Autodesk Fusion 360 part; units mm, degrees
(part 4 of 5)
  spline S13 degree 5 poles (13.9862, 0.6207) (13.9784, 0.6259) (13.9629, 0.6363) (13.9395, 0.6518) (13.9082, 0.6724) (13.8691, 0.6978) (13.8299, 0.7229) (13.7907, 0.7477) (13.7514, 0.7723) (13.712, 0.7966) (13.6725, 0.8206) (13.633, 0.8443) (13.5934, 0.8678) (13.5538, 0.8909) (13.514, 0.9138) (13.4743, 0.9364) (13.4344, 0.9587) (13.3946, 0.9807) (13.3546, 1.0024) (13.3146, 1.0239) (13.2746, 1.045) (13.2345, 1.0658) (13.1943, 1.0863) (13.1541, 1.1066) (13.1138, 1.1265) (13.0735, 1.1461) (13.0332, 1.1654) (12.9928, 1.1844) (12.9523, 1.2031) (12.9119, 1.2215) (12.8713, 1.2395) (12.8308, 1.2572) (12.7902, 1.2746) (12.7495, 1.2917) (12.7088, 1.3084) (12.6681, 1.3248) (12.6274, 1.3409) (12.5866, 1.3566) (12.5458, 1.372) (12.505, 1.3871) (12.4641, 1.4018) (12.4233, 1.4161) (12.3824, 1.4301) (12.3414, 1.4437) (12.3005, 1.4569) (12.2595, 1.4698) (12.2186, 1.4823) (12.1776, 1.4944) (12.1366, 1.5062) (12.0956, 1.5175) (12.0545, 1.5285) (12.0135, 1.539) (11.9725, 1.5491) (11.9315, 1.5587) (11.8905, 1.5678) (11.8494, 1.5766) (11.8084, 1.585) (11.7674, 1.5929) (11.7264, 1.6005) (11.6854, 1.6075) (11.6445, 1.614) (11.6035, 1.6199) (11.5626, 1.625) (11.5218, 1.6295) (11.4809, 1.6333) (11.4401, 1.6366) (11.3994, 1.6396) (11.3587, 1.6423) (11.318, 1.6445) (11.2774, 1.6458) (11.237, 1.6456) (11.2048, 1.6439) (11.1807, 1.6416) (11.1647, 1.6395) (11.1567, 1.6383) knots -1 -1 -1 -1 -1 -1 -0.98571429 -0.97142857 -0.95714286 -0.94285714 -0.92857143 -0.91428571 -0.9 -0.88571429 -0.87142857 -0.85714286 -0.84285714 -0.82857143 -0.81428571 -0.8 -0.78571429 -0.77142857 -0.75714286 -0.74285714 -0.72857143 -0.71428571 -0.7 -0.68571429 -0.67142857 -0.65714286 -0.64285714 -0.62857143 -0.61428571 -0.6 -0.58571429 -0.57142857 -0.55714286 -0.54285714 -0.52857143 -0.51428571 -0.5 -0.48571429 -0.47142857 -0.45714286 -0.44285714 -0.42857143 -0.41428571 -0.4 -0.38571429 -0.37142857 -0.35714286 -0.34285714 -0.32857143 -0.31428571 -0.3 -0.28571429 -0.27142857 -0.25714286 -0.24285714 -0.22857143 -0.21428571 -0.2 -0.18571429 -0.17142857 -0.15714286 -0.14285714 -0.12857143 -0.11428571 -0.1 -0.08571429 -0.07142857 -0.05714286 -0.04285714 -0.02857143 -0.01428571 0 0 0 0 0 0
  line L13 (11.1567, 1.6383) -> (10.3893, 1.5263)
  arc A27 (9.2737, 2.2773) -> (10.3893, 1.5263) centre (10.2448, 2.5158) ccw
  arc A28 (9.2737, 2.2773) -> (9.1699, 2.6646) centre (0, 0) ccw
  arc A29 (9.7605, 3.8729) -> (9.1699, 2.6646) centre (10.1302, 2.9437) ccw
  line L14 (9.7605, 3.8729) -> (10.4811, 4.1595)
  spline S14 degree 5 poles (10.4811, 4.1595) (10.4886, 4.1625) (10.5035, 4.1687) (10.5256, 4.1787) (10.5543, 4.1933) (10.5894, 4.2134) (10.6239, 4.2349) (10.658, 4.2571) (10.692, 4.2797) (10.7258, 4.3027) (10.7594, 4.326) (10.7929, 4.3497) (10.826, 4.374) (10.8589, 4.3989) (10.8914, 4.4244) (10.9236, 4.4505) (10.9556, 4.4772) (10.9873, 4.5042) (11.0189, 4.5316) (11.0502, 4.5593) (11.0814, 4.5874) (11.1123, 4.6159) (11.143, 4.6447) (11.1735, 4.674) (11.2038, 4.7036) (11.2338, 4.7336) (11.2637, 4.7639) (11.2933, 4.7946) (11.3227, 4.8256) (11.352, 4.8569) (11.381, 4.8885) (11.4099, 4.9204) (11.4385, 4.9527) (11.4669, 4.9852) (11.4952, 5.0181) (11.5232, 5.0512) (11.551, 5.0847) (11.5787, 5.1184) (11.6061, 5.1524) (11.6334, 5.1867) (11.6604, 5.2213) (11.6873, 5.2561) (11.7139, 5.2912) (11.7404, 5.3266) (11.7666, 5.3622) (11.7927, 5.3981) (11.8186, 5.4343) (11.8443, 5.4707) (11.8698, 5.5073) (11.8951, 5.5442) (11.9202, 5.5813) (11.9451, 5.6187) (11.9698, 5.6563) (11.9943, 5.6942) (12.0186, 5.7323) (12.0427, 5.7706) (12.0667, 5.8092) (12.0904, 5.848) (12.1139, 5.887) (12.1373, 5.9262) (12.1604, 5.9656) (12.1834, 6.0053) (12.2061, 6.0452) (12.2287, 6.0853) (12.251, 6.1256) (12.2732, 6.1661) (12.2952, 6.2069) (12.3169, 6.2478) (12.3385, 6.2889) (12.3599, 6.3303) (12.3811, 6.3718) (12.3979, 6.4052) (12.4104, 6.4304) (12.4186, 6.4472) (12.4228, 6.4556) knots 0 0 0 0 0 0 0.01428571 0.02857143 0.04285714 0.05714286 0.07142857 0.08571429 0.1 0.11428571 0.12857143 0.14285714 0.15714286 0.17142857 0.18571429 0.2 0.21428571 0.22857143 0.24285714 0.25714286 0.27142857 0.28571429 0.3 0.31428571 0.32857143 0.34285714 0.35714286 0.37142857 0.38571429 0.4 0.41428571 0.42857143 0.44285714 0.45714286 0.47142857 0.48571429 0.5 0.51428571 0.52857143 0.54285714 0.55714286 0.57142857 0.58571429 0.6 0.61428571 0.62857143 0.64285714 0.65714286 0.67142857 0.68571429 0.7 0.71428571 0.72857143 0.74285714 0.75714286 0.77142857 0.78571429 0.8 0.81428571 0.82857143 0.84285714 0.85714286 0.87142857 0.88571429 0.9 0.91428571 0.92857143 0.94285714 0.95714286 0.97142857 0.98571429 1 1 1 1 1 1
  arc A30 (12.4228, 6.4556) -> (11.8021, 7.5307) centre (0, 0) ccw
  spline S15 degree 5 poles (11.8021, 7.5307) (11.7927, 7.5313) (11.774, 7.5325) (11.746, 7.5342) (11.7087, 7.5364) (11.6621, 7.5388) (11.6156, 7.541) (11.5692, 7.5429) (11.5229, 7.5445) (11.4766, 7.5458) (11.4305, 7.5469) (11.3844, 7.5477) (11.3384, 7.5482) (11.2924, 7.5484) (11.2466, 7.5484) (11.2009, 7.5481) (11.1552, 7.5475) (11.1097, 7.5466) (11.0642, 7.5454) (11.0189, 7.544) (10.9736, 7.5423) (10.9285, 7.5403) (10.8834, 7.538) (10.8385, 7.5354) (10.7937, 7.5325) (10.7489, 7.5293) (10.7044, 7.5259) (10.6599, 7.5221) (10.6155, 7.5181) (10.5713, 7.5137) (10.5271, 7.5091) (10.4832, 7.5042) (10.4393, 7.4989) (10.3956, 7.4934) (10.352, 7.4876) (10.3085, 7.4814) (10.2652, 7.475) (10.222, 7.4682) (10.179, 7.4611) (10.1361, 7.4538) (10.0934, 7.4461) (10.0508, 7.438) (10.0084, 7.4297) (9.9662, 7.421) (9.9241, 7.412) (9.8822, 7.4027) (9.8404, 7.393) (9.7989, 7.383) (9.7575, 7.3727) (9.7163, 7.362) (9.6753, 7.351) (9.6345, 7.3396) (9.594, 7.3278) (9.5536, 7.3156) (9.5135, 7.303) (9.4736, 7.2901) (9.4339, 7.2768) (9.3944, 7.2632) (9.3551, 7.2492) (9.3161, 7.2349) (9.2774, 7.22) (9.239, 7.2046) (9.201, 7.1886) (9.1634, 7.172) (9.1261, 7.1549) (9.0891, 7.1374) (9.0523, 7.1196) (9.0157, 7.1016) (8.9794, 7.0831) (8.9437, 7.064) (8.9087, 7.0436) (8.8816, 7.0261) (8.862, 7.012) (8.8491, 7.0022) (8.8428, 6.9972) knots -1 -1 -1 -1 -1 -1 -0.98571429 -0.97142857 -0.95714286 -0.94285714 -0.92857143 -0.91428571 -0.9 -0.88571429 -0.87142857 -0.85714286 -0.84285714 -0.82857143 -0.81428571 -0.8 -0.78571429 -0.77142857 -0.75714286 -0.74285714 -0.72857143 -0.71428571 -0.7 -0.68571429 -0.67142857 -0.65714286 -0.64285714 -0.62857143 -0.61428571 -0.6 -0.58571429 -0.57142857 -0.55714286 -0.54285714 -0.52857143 -0.51428571 -0.5 -0.48571429 -0.47142857 -0.45714286 -0.44285714 -0.42857143 -0.41428571 -0.4 -0.38571429 -0.37142857 -0.35714286 -0.34285714 -0.32857143 -0.31428571 -0.3 -0.28571429 -0.27142857 -0.25714286 -0.24285714 -0.22857143 -0.21428571 -0.2 -0.18571429 -0.17142857 -0.15714286 -0.14285714 -0.12857143 -0.11428571 -0.1 -0.08571429 -0.07142857 -0.05714286 -0.04285714 -0.02857143 -0.01428571 0 0 0 0 0 0
  line L15 (8.8428, 6.9972) -> (8.2343, 6.5164)
  arc A31 (6.8926, 6.609) -> (8.2343, 6.5164) centre (7.6144, 7.3011) ccw
  arc A32 (6.8926, 6.609) -> (6.609, 6.8926) centre (0, 0) ccw
  arc A33 (6.5164, 8.2343) -> (6.609, 6.8926) centre (7.3011, 7.6144) ccw
  line L16 (6.5164, 8.2343) -> (6.9972, 8.8428)
  spline S16 degree 5 poles (6.9972, 8.8428) (7.0022, 8.8491) (7.012, 8.862) (7.0261, 8.8816) (7.0436, 8.9087) (7.064, 8.9437) (7.0831, 8.9794) (7.1016, 9.0157) (7.1196, 9.0523) (7.1374, 9.0891) (7.1549, 9.1261) (7.172, 9.1634) (7.1886, 9.201) (7.2046, 9.239) (7.22, 9.2774) (7.2349, 9.3161) (7.2492, 9.3551) (7.2632, 9.3944) (7.2768, 9.4339) (7.2901, 9.4736) (7.303, 9.5135) (7.3156, 9.5536) (7.3278, 9.594) (7.3396, 9.6345) (7.351, 9.6753) (7.362, 9.7163) (7.3727, 9.7575) (7.383, 9.7989) (7.393, 9.8404) (7.4027, 9.8822) (7.412, 9.9241) (7.421, 9.9662) (7.4297, 10.0084) (7.438, 10.0508) (7.4461, 10.0934) (7.4538, 10.1361) (7.4611, 10.179) (7.4682, 10.222) (7.475, 10.2652) (7.4814, 10.3085) (7.4876, 10.352) (7.4934, 10.3956) (7.4989, 10.4393) (7.5042, 10.4832) (7.5091, 10.5271) (7.5137, 10.5713) (7.5181, 10.6155) (7.5221, 10.6599) (7.5259, 10.7044) (7.5293, 10.7489) (7.5325, 10.7937) (7.5354, 10.8385) (7.538, 10.8834) (7.5403, 10.9285) (7.5423, 10.9736) (7.544, 11.0189) (7.5454, 11.0642) (7.5466, 11.1097) (7.5475, 11.1552) (7.5481, 11.2009) (7.5484, 11.2466) (7.5484, 11.2924) (7.5482, 11.3384) (7.5477, 11.3844) (7.5469, 11.4305) (7.5458, 11.4766) (7.5445, 11.5229) (7.5429, 11.5692) (7.541, 11.6156) (7.5388, 11.6621) (7.5364, 11.7087) (7.5342, 11.746) (7.5325, 11.774) (7.5313, 11.7927) (7.5307, 11.8021) knots 0 0 0 0 0 0 0.01428571 0.02857143 0.04285714 0.05714286 0.07142857 0.08571429 0.1 0.11428571 0.12857143 0.14285714 0.15714286 0.17142857 0.18571429 0.2 0.21428571 0.22857143 0.24285714 0.25714286 0.27142857 0.28571429 0.3 0.31428571 0.32857143 0.34285714 0.35714286 0.37142857 0.38571429 0.4 0.41428571 0.42857143 0.44285714 0.45714286 0.47142857 0.48571429 0.5 0.51428571 0.52857143 0.54285714 0.55714286 0.57142857 0.58571429 0.6 0.61428571 0.62857143 0.64285714 0.65714286 0.67142857 0.68571429 0.7 0.71428571 0.72857143 0.74285714 0.75714286 0.77142857 0.78571429 0.8 0.81428571 0.82857143 0.84285714 0.85714286 0.87142857 0.88571429 0.9 0.91428571 0.92857143 0.94285714 0.95714286 0.97142857 0.98571429 1 1 1 1 1 1
  arc A34 (7.5307, 11.8021) -> (6.4556, 12.4228) centre (0, 0) ccw
  spline S17 degree 5 poles (6.4556, 12.4228) (6.4472, 12.4186) (6.4304, 12.4104) (6.4052, 12.3979) (6.3718, 12.3811) (6.3303, 12.3599) (6.2889, 12.3385) (6.2478, 12.3169) (6.2069, 12.2952) (6.1661, 12.2732) (6.1256, 12.251) (6.0853, 12.2287) (6.0452, 12.2061) (6.0053, 12.1834) (5.9656, 12.1604) (5.9262, 12.1373) (5.887, 12.1139) (5.848, 12.0904) (5.8092, 12.0667) (5.7706, 12.0427) (5.7323, 12.0186) (5.6942, 11.9943) (5.6563, 11.9698) (5.6187, 11.9451) (5.5813, 11.9202) (5.5442, 11.8951) (5.5073, 11.8698) (5.4707, 11.8443) (5.4343, 11.8186) (5.3981, 11.7927) (5.3622, 11.7666) (5.3266, 11.7404) (5.2912, 11.7139) (5.2561, 11.6873) (5.2213, 11.6604) (5.1867, 11.6334) (5.1524, 11.6061) (5.1184, 11.5787) (5.0847, 11.551) (5.0512, 11.5232) (5.0181, 11.4952) (4.9852, 11.4669) (4.9527, 11.4385) (4.9204, 11.4099) (4.8885, 11.381) (4.8569, 11.352) (4.8256, 11.3227) (4.7946, 11.2933) (4.7639, 11.2637) (4.7336, 11.2338) (4.7036, 11.2038) (4.674, 11.1735) (4.6447, 11.143) (4.6159, 11.1123) (4.5874, 11.0814) (4.5593, 11.0502) (4.5316, 11.0189) (4.5042, 10.9873) (4.4772, 10.9556) (4.4505, 10.9236) (4.4244, 10.8914) (4.3989, 10.8589) (4.374, 10.826) (4.3497, 10.7929) (4.326, 10.7594) (4.3027, 10.7258) (4.2797, 10.692) (4.2571, 10.658) (4.2349, 10.6239) (4.2134, 10.5894) (4.1933, 10.5543) (4.1787, 10.5256) (4.1687, 10.5035) (4.1625, 10.4886) (4.1595, 10.4811) knots -1 -1 -1 -1 -1 -1 -0.98571429 -0.97142857 -0.95714286 -0.94285714 -0.92857143 -0.91428571 -0.9 -0.88571429 -0.87142857 -0.85714286 -0.84285714 -0.82857143 -0.81428571 -0.8 -0.78571429 -0.77142857 -0.75714286 -0.74285714 -0.72857143 -0.71428571 -0.7 -0.68571429 -0.67142857 -0.65714286 -0.64285714 -0.62857143 -0.61428571 -0.6 -0.58571429 -0.57142857 -0.55714286 -0.54285714 -0.52857143 -0.51428571 -0.5 -0.48571429 -0.47142857 -0.45714286 -0.44285714 -0.42857143 -0.41428571 -0.4 -0.38571429 -0.37142857 -0.35714286 -0.34285714 -0.32857143 -0.31428571 -0.3 -0.28571429 -0.27142857 -0.25714286 -0.24285714 -0.22857143 -0.21428571 -0.2 -0.18571429 -0.17142857 -0.15714286 -0.14285714 -0.12857143 -0.11428571 -0.1 -0.08571429 -0.07142857 -0.05714286 -0.04285714 -0.02857143 -0.01428571 0 0 0 0 0 0
  line L17 (4.1595, 10.4811) -> (3.8729, 9.7605)
  arc A35 (2.6646, 9.1699) -> (3.8729, 9.7605) centre (2.9437, 10.1302) ccw
  arc A36 (2.6646, 9.1699) -> (2.2773, 9.2737) centre (0, 0) ccw
  arc A37 (1.5263, 10.3893) -> (2.2773, 9.2737) centre (2.5158, 10.2448) ccw
  line L18 (1.5263, 10.3893) -> (1.6383, 11.1567)
  spline S18 degree 5 poles (1.6383, 11.1567) (1.6395, 11.1647) (1.6416, 11.1807) (1.6439, 11.2048) (1.6456, 11.237) (1.6458, 11.2774) (1.6445, 11.318) (1.6423, 11.3587) (1.6396, 11.3994) (1.6366, 11.4401) (1.6333, 11.4809) (1.6295, 11.5218) (1.625, 11.5626) (1.6199, 11.6035) (1.614, 11.6445) (1.6075, 11.6854) (1.6005, 11.7264) (1.5929, 11.7674) (1.585, 11.8084) (1.5766, 11.8494) (1.5678, 11.8905) (1.5587, 11.9315) (1.5491, 11.9725) (1.539, 12.0135) (1.5285, 12.0545) (1.5175, 12.0956) (1.5062, 12.1366) (1.4944, 12.1776) (1.4823, 12.2186) (1.4698, 12.2595) (1.4569, 12.3005) (1.4437, 12.3414) (1.4301, 12.3824) (1.4161, 12.4233) (1.4018, 12.4641) (1.3871, 12.505) (1.372, 12.5458) (1.3566, 12.5866) (1.3409, 12.6274) (1.3248, 12.6681) (1.3084, 12.7088) (1.2917, 12.7495) (1.2746, 12.7902) (1.2572, 12.8308) (1.2395, 12.8713) (1.2215, 12.9119) (1.2031, 12.9523) (1.1844, 12.9928) (1.1654, 13.0332) (1.1461, 13.0735) (1.1265, 13.1138) (1.1066, 13.1541) (1.0863, 13.1943) (1.0658, 13.2345) (1.045, 13.2746) (1.0239, 13.3146) (1.0024, 13.3546) (0.9807, 13.3946) (0.9587, 13.4344) (0.9364, 13.4743) (0.9138, 13.514) (0.8909, 13.5538) (0.8678, 13.5934) (0.8443, 13.633) (0.8206, 13.6725) (0.7966, 13.712) (0.7723, 13.7514) (0.7477, 13.7907) (0.7229, 13.8299) (0.6978, 13.8691) (0.6724, 13.9082) (0.6518, 13.9395) (0.6363, 13.9629) (0.6259, 13.9784) (0.6207, 13.9862) knots 0 0 0 0 0 0 0.01428571 0.02857143 0.04285714 0.05714286 0.07142857 0.08571429 0.1 0.11428571 0.12857143 0.14285714 0.15714286 0.17142857 0.18571429 0.2 0.21428571 0.22857143 0.24285714 0.25714286 0.27142857 0.28571429 0.3 0.31428571 0.32857143 0.34285714 0.35714286 0.37142857 0.38571429 0.4 0.41428571 0.42857143 0.44285714 0.45714286 0.47142857 0.48571429 0.5 0.51428571 0.52857143 0.54285714 0.55714286 0.57142857 0.58571429 0.6 0.61428571 0.62857143 0.64285714 0.65714286 0.67142857 0.68571429 0.7 0.71428571 0.72857143 0.74285714 0.75714286 0.77142857 0.78571429 0.8 0.81428571 0.82857143 0.84285714 0.85714286 0.87142857 0.88571429 0.9 0.91428571 0.92857143 0.94285714 0.95714286 0.97142857 0.98571429 1 1 1 1 1 1
  arc A38 (0.6207, 13.9862) -> (-0.6207, 13.9862) centre (0, 0) ccw
  spline S19 degree 5 poles (-0.6207, 13.9862) (-0.6259, 13.9784) (-0.6363, 13.9629) (-0.6518, 13.9395) (-0.6724, 13.9082) (-0.6978, 13.8691) (-0.7229, 13.8299) (-0.7477, 13.7907) (-0.7723, 13.7514) (-0.7966, 13.712) (-0.8206, 13.6725) (-0.8443, 13.633) (-0.8678, 13.5934) (-0.8909, 13.5538) (-0.9138, 13.514) (-0.9364, 13.4743) (-0.9587, 13.4344) (-0.9807, 13.3946) (-1.0024, 13.3546) (-1.0239, 13.3146) (-1.045, 13.2746) (-1.0658, 13.2345) (-1.0863, 13.1943) (-1.1066, 13.1541) (-1.1265, 13.1138) (-1.1461, 13.0735) (-1.1654, 13.0332) (-1.1844, 12.9928) (-1.2031, 12.9523) (-1.2215, 12.9119) (-1.2395, 12.8713) (-1.2572, 12.8308) (-1.2746, 12.7902) (-1.2917, 12.7495) (-1.3084, 12.7088) (-1.3248, 12.6681) (-1.3409, 12.6274) (-1.3566, 12.5866) (-1.372, 12.5458) (-1.3871, 12.505) (-1.4018, 12.4641) (-1.4161, 12.4233) (-1.4301, 12.3824) (-1.4437, 12.3414) (-1.4569, 12.3005) (-1.4698, 12.2595) (-1.4823, 12.2186) (-1.4944, 12.1776) (-1.5062, 12.1366) (-1.5175, 12.0956) (-1.5285, 12.0545) (-1.539, 12.0135) (-1.5491, 11.9725) (-1.5587, 11.9315) (-1.5678, 11.8905) (-1.5766, 11.8494) (-1.585, 11.8084) (-1.5929, 11.7674) (-1.6005, 11.7264) (-1.6075, 11.6854) (-1.614, 11.6445) (-1.6199, 11.6035) (-1.625, 11.5626) (-1.6295, 11.5218) (-1.6333, 11.4809) (-1.6366, 11.4401) (-1.6396, 11.3994) (-1.6423, 11.3587) (-1.6445, 11.318) (-1.6458, 11.2774) (-1.6456, 11.237) (-1.6439, 11.2048) (-1.6416, 11.1807) (-1.6395, 11.1647) (-1.6383, 11.1567) knots -1 -1 -1 -1 -1 -1 -0.98571429 -0.97142857 -0.95714286 -0.94285714 -0.92857143 -0.91428571 -0.9 -0.88571429 -0.87142857 -0.85714286 -0.84285714 -0.82857143 -0.81428571 -0.8 -0.78571429 -0.77142857 -0.75714286 -0.74285714 -0.72857143 -0.71428571 -0.7 -0.68571429 -0.67142857 -0.65714286 -0.64285714 -0.62857143 -0.61428571 -0.6 -0.58571429 -0.57142857 -0.55714286 -0.54285714 -0.52857143 -0.51428571 -0.5 -0.48571429 -0.47142857 -0.45714286 -0.44285714 -0.42857143 -0.41428571 -0.4 -0.38571429 -0.37142857 -0.35714286 -0.34285714 -0.32857143 -0.31428571 -0.3 -0.28571429 -0.27142857 -0.25714286 -0.24285714 -0.22857143 -0.21428571 -0.2 -0.18571429 -0.17142857 -0.15714286 -0.14285714 -0.12857143 -0.11428571 -0.1 -0.08571429 -0.07142857 -0.05714286 -0.04285714 -0.02857143 -0.01428571 0 0 0 0 0 0
  line L19 (-1.6383, 11.1567) -> (-1.5263, 10.3893)
  arc A39 (-2.2773, 9.2737) -> (-1.5263, 10.3893) centre (-2.5158, 10.2448) ccw
  arc A40 (-2.2773, 9.2737) -> (-2.6646, 9.1699) centre (0, 0) ccw
  arc A41 (-3.8729, 9.7605) -> (-2.6646, 9.1699) centre (-2.9437, 10.1302) ccw
  line L20 (-3.8729, 9.7605) -> (-4.1595, 10.4811)
  spline S20 degree 5 poles (-4.1595, 10.4811) (-4.1625, 10.4886) (-4.1687, 10.5035) (-4.1787, 10.5256) (-4.1933, 10.5543) (-4.2134, 10.5894) (-4.2349, 10.6239) (-4.2571, 10.658) (-4.2797, 10.692) (-4.3027, 10.7258) (-4.326, 10.7594) (-4.3497, 10.7929) (-4.374, 10.826) (-4.3989, 10.8589) (-4.4244, 10.8914) (-4.4505, 10.9236) (-4.4772, 10.9556) (-4.5042, 10.9873) (-4.5316, 11.0189) (-4.5593, 11.0502) (-4.5874, 11.0814) (-4.6159, 11.1123) (-4.6447, 11.143) (-4.674, 11.1735) (-4.7036, 11.2038) (-4.7336, 11.2338) (-4.7639, 11.2637) (-4.7946, 11.2933) (-4.8256, 11.3227) (-4.8569, 11.352) (-4.8885, 11.381) (-4.9204, 11.4099) (-4.9527, 11.4385) (-4.9852, 11.4669) (-5.0181, 11.4952) (-5.0512, 11.5232) (-5.0847, 11.551) (-5.1184, 11.5787) (-5.1524, 11.6061) (-5.1867, 11.6334) (-5.2213, 11.6604) (-5.2561, 11.6873) (-5.2912, 11.7139) (-5.3266, 11.7404) (-5.3622, 11.7666) (-5.3981, 11.7927) (-5.4343, 11.8186) (-5.4707, 11.8443) (-5.5073, 11.8698) (-5.5442, 11.8951) (-5.5813, 11.9202) (-5.6187, 11.9451) (-5.6563, 11.9698) (-5.6942, 11.9943) (-5.7323, 12.0186) (-5.7706, 12.0427) (-5.8092, 12.0667) (-5.848, 12.0904) (-5.887, 12.1139) (-5.9262, 12.1373) (-5.9656, 12.1604) (-6.0053, 12.1834) (-6.0452, 12.2061) (-6.0853, 12.2287) (-6.1256, 12.251) (-6.1661, 12.2732) (-6.2069, 12.2952) (-6.2478, 12.3169) (-6.2889, 12.3385) (-6.3303, 12.3599) (-6.3718, 12.3811) (-6.4052, 12.3979) (-6.4304, 12.4104) (-6.4472, 12.4186) (-6.4556, 12.4228) knots 0 0 0 0 0 0 0.01428571 0.02857143 0.04285714 0.05714286 0.07142857 0.08571429 0.1 0.11428571 0.12857143 0.14285714 0.15714286 0.17142857 0.18571429 0.2 0.21428571 0.22857143 0.24285714 0.25714286 0.27142857 0.28571429 0.3 0.31428571 0.32857143 0.34285714 0.35714286 0.37142857 0.38571429 0.4 0.41428571 0.42857143 0.44285714 0.45714286 0.47142857 0.48571429 0.5 0.51428571 0.52857143 0.54285714 0.55714286 0.57142857 0.58571429 0.6 0.61428571 0.62857143 0.64285714 0.65714286 0.67142857 0.68571429 0.7 0.71428571 0.72857143 0.74285714 0.75714286 0.77142857 0.78571429 0.8 0.81428571 0.82857143 0.84285714 0.85714286 0.87142857 0.88571429 0.9 0.91428571 0.92857143 0.94285714 0.95714286 0.97142857 0.98571429 1 1 1 1 1 1
  arc A42 (-6.4556, 12.4228) -> (-7.5307, 11.8021) centre (0, 0) ccw
  spline S21 degree 5 poles (-7.5307, 11.8021) (-7.5313, 11.7927) (-7.5325, 11.774) (-7.5342, 11.746) (-7.5364, 11.7087) (-7.5388, 11.6621) (-7.541, 11.6156) (-7.5429, 11.5692) (-7.5445, 11.5229) (-7.5458, 11.4766) (-7.5469, 11.4305) (-7.5477, 11.3844) (-7.5482, 11.3384) (-7.5484, 11.2924) (-7.5484, 11.2466) (-7.5481, 11.2009) (-7.5475, 11.1552) (-7.5466, 11.1097) (-7.5454, 11.0642) (-7.544, 11.0189) (-7.5423, 10.9736) (-7.5403, 10.9285) (-7.538, 10.8834) (-7.5354, 10.8385) (-7.5325, 10.7937) (-7.5293, 10.7489) (-7.5259, 10.7044) (-7.5221, 10.6599) (-7.5181, 10.6155) (-7.5137, 10.5713) (-7.5091, 10.5271) (-7.5042, 10.4832) (-7.4989, 10.4393) (-7.4934, 10.3956) (-7.4876, 10.352) (-7.4814, 10.3085) (-7.475, 10.2652) (-7.4682, 10.222) (-7.4611, 10.179) (-7.4538, 10.1361) (-7.4461, 10.0934) (-7.438, 10.0508) (-7.4297, 10.0084) (-7.421, 9.9662) (-7.412, 9.9241) (-7.4027, 9.8822) (-7.393, 9.8404) (-7.383, 9.7989) (-7.3727, 9.7575) (-7.362, 9.7163) (-7.351, 9.6753) (-7.3396, 9.6345) (-7.3278, 9.594) (-7.3156, 9.5536) (-7.303, 9.5135) (-7.2901, 9.4736) (-7.2768, 9.4339) (-7.2632, 9.3944) (-7.2492, 9.3551) (-7.2349, 9.3161) (-7.22, 9.2774) (-7.2046, 9.239) (-7.1886, 9.201) (-7.172, 9.1634) (-7.1549, 9.1261) (-7.1374, 9.0891) (-7.1196, 9.0523) (-7.1016, 9.0157) (-7.0831, 8.9794) (-7.064, 8.9437) (-7.0436, 8.9087) (-7.0261, 8.8816) (-7.012, 8.862) (-7.0022, 8.8491) (-6.9972, 8.8428) knots -1 -1 -1 -1 -1 -1 -0.98571429 -0.97142857 -0.95714286 -0.94285714 -0.92857143 -0.91428571 -0.9 -0.88571429 -0.87142857 -0.85714286 -0.84285714 -0.82857143 -0.81428571 -0.8 -0.78571429 -0.77142857 -0.75714286 -0.74285714 -0.72857143 -0.71428571 -0.7 -0.68571429 -0.67142857 -0.65714286 -0.64285714 -0.62857143 -0.61428571 -0.6 -0.58571429 -0.57142857 -0.55714286 -0.54285714 -0.52857143 -0.51428571 -0.5 -0.48571429 -0.47142857 -0.45714286 -0.44285714 -0.42857143 -0.41428571 -0.4 -0.38571429 -0.37142857 -0.35714286 -0.34285714 -0.32857143 -0.31428571 -0.3 -0.28571429 -0.27142857 -0.25714286 -0.24285714 -0.22857143 -0.21428571 -0.2 -0.18571429 -0.17142857 -0.15714286 -0.14285714 -0.12857143 -0.11428571 -0.1 -0.08571429 -0.07142857 -0.05714286 -0.04285714 -0.02857143 -0.01428571 0 0 0 0 0 0
  line L21 (-6.9972, 8.8428) -> (-6.5164, 8.2343)
  arc A43 (-6.609, 6.8926) -> (-6.5164, 8.2343) centre (-7.3011, 7.6144) ccw
  arc A44 (-6.609, 6.8926) -> (-6.8926, 6.609) centre (0, 0) ccw
  arc A45 (-8.2343, 6.5164) -> (-6.8926, 6.609) centre (-7.6144, 7.3011) ccw
  line L22 (-8.2343, 6.5164) -> (-8.8428, 6.9972)
  spline S22 degree 5 poles (-8.8428, 6.9972) (-8.8491, 7.0022) (-8.862, 7.012) (-8.8816, 7.0261) (-8.9087, 7.0436) (-8.9437, 7.064) (-8.9794, 7.0831) (-9.0157, 7.1016) (-9.0523, 7.1196) (-9.0891, 7.1374) (-9.1261, 7.1549) (-9.1634, 7.172) (-9.201, 7.1886) (-9.239, 7.2046) (-9.2774, 7.22) (-9.3161, 7.2349) (-9.3551, 7.2492) (-9.3944, 7.2632) (-9.4339, 7.2768) (-9.4736, 7.2901) (-9.5135, 7.303) (-9.5536, 7.3156) (-9.594, 7.3278) (-9.6345, 7.3396) (-9.6753, 7.351) (-9.7163, 7.362) (-9.7575, 7.3727) (-9.7989, 7.383) (-9.8404, 7.393) (-9.8822, 7.4027) (-9.9241, 7.412) (-9.9662, 7.421) (-10.0084, 7.4297) (-10.0508, 7.438) (-10.0934, 7.4461) (-10.1361, 7.4538) (-10.179, 7.4611) (-10.222, 7.4682) (-10.2652, 7.475) (-10.3085, 7.4814) (-10.352, 7.4876) (-10.3956, 7.4934) (-10.4393, 7.4989) (-10.4832, 7.5042) (-10.5271, 7.5091) (-10.5713, 7.5137) (-10.6155, 7.5181) (-10.6599, 7.5221) (-10.7044, 7.5259) (-10.7489, 7.5293) (-10.7937, 7.5325) (-10.8385, 7.5354) (-10.8834, 7.538) (-10.9285, 7.5403) (-10.9736, 7.5423) (-11.0189, 7.544) (-11.0642, 7.5454) (-11.1097, 7.5466) (-11.1552, 7.5475) (-11.2009, 7.5481) (-11.2466, 7.5484) (-11.2924, 7.5484) (-11.3384, 7.5482) (-11.3844, 7.5477) (-11.4305, 7.5469) (-11.4766, 7.5458) (-11.5229, 7.5445) (-11.5692, 7.5429) (-11.6156, 7.541) (-11.6621, 7.5388) (-11.7087, 7.5364) (-11.746, 7.5342) (-11.774, 7.5325) (-11.7927, 7.5313) (-11.8021, 7.5307) knots 0 0 0 0 0 0 0.01428571 0.02857143 0.04285714 0.05714286 0.07142857 0.08571429 0.1 0.11428571 0.12857143 0.14285714 0.15714286 0.17142857 0.18571429 0.2 0.21428571 0.22857143 0.24285714 0.25714286 0.27142857 0.28571429 0.3 0.31428571 0.32857143 0.34285714 0.35714286 0.37142857 0.38571429 0.4 0.41428571 0.42857143 0.44285714 0.45714286 0.47142857 0.48571429 0.5 0.51428571 0.52857143 0.54285714 0.55714286 0.57142857 0.58571429 0.6 0.61428571 0.62857143 0.64285714 0.65714286 0.67142857 0.68571429 0.7 0.71428571 0.72857143 0.74285714 0.75714286 0.77142857 0.78571429 0.8 0.81428571 0.82857143 0.84285714 0.85714286 0.87142857 0.88571429 0.9 0.91428571 0.92857143 0.94285714 0.95714286 0.97142857 0.98571429 1 1 1 1 1 1
  arc A46 (-11.8021, 7.5307) -> (-12.4228, 6.4556) centre (0, 0) ccw
  spline S23 degree 5 poles (-12.4228, 6.4556) (-12.4186, 6.4472) (-12.4104, 6.4304) (-12.3979, 6.4052) (-12.3811, 6.3718) (-12.3599, 6.3303) (-12.3385, 6.2889) (-12.3169, 6.2478) (-12.2952, 6.2069) (-12.2732, 6.1661) (-12.251, 6.1256) (-12.2287, 6.0853) (-12.2061, 6.0452) (-12.1834, 6.0053) (-12.1604, 5.9656) (-12.1373, 5.9262) (-12.1139, 5.887) (-12.0904, 5.848) (-12.0667, 5.8092) (-12.0427, 5.7706) (-12.0186, 5.7323) (-11.9943, 5.6942) (-11.9698, 5.6563) (-11.9451, 5.6187) (-11.9202, 5.5813) (-11.8951, 5.5442) (-11.8698, 5.5073) (-11.8443, 5.4707) (-11.8186, 5.4343) (-11.7927, 5.3981) (-11.7666, 5.3622) (-11.7404, 5.3266) (-11.7139, 5.2912) (-11.6873, 5.2561) (-11.6604, 5.2213) (-11.6334, 5.1867) (-11.6061, 5.1524) (-11.5787, 5.1184) (-11.551, 5.0847) (-11.5232, 5.0512) (-11.4952, 5.0181) (-11.4669, 4.9852) (-11.4385, 4.9527) (-11.4099, 4.9204) (-11.381, 4.8885) (-11.352, 4.8569) (-11.3227, 4.8256) (-11.2933, 4.7946) (-11.2637, 4.7639) (-11.2338, 4.7336) (-11.2038, 4.7036) (-11.1735, 4.674) (-11.143, 4.6447) (-11.1123, 4.6159) (-11.0814, 4.5874) (-11.0502, 4.5593) (-11.0189, 4.5316) (-10.9873, 4.5042) (-10.9556, 4.4772) (-10.9236, 4.4505) (-10.8914, 4.4244) (-10.8589, 4.3989) (-10.826, 4.374) (-10.7929, 4.3497) (-10.7594, 4.326) (-10.7258, 4.3027) (-10.692, 4.2797) (-10.658, 4.2571) (-10.6239, 4.2349) (-10.5894, 4.2134) (-10.5543, 4.1933) (-10.5256, 4.1787) (-10.5035, 4.1687) (-10.4886, 4.1625) (-10.4811, 4.1595) knots -1 -1 -1 -1 -1 -1 -0.98571429 -0.97142857 -0.95714286 -0.94285714 -0.92857143 -0.91428571 -0.9 -0.88571429 -0.87142857 -0.85714286 -0.84285714 -0.82857143 -0.81428571 -0.8 -0.78571429 -0.77142857 -0.75714286 -0.74285714 -0.72857143 -0.71428571 -0.7 -0.68571429 -0.67142857 -0.65714286 -0.64285714 -0.62857143 -0.61428571 -0.6 -0.58571429 -0.57142857 -0.55714286 -0.54285714 -0.52857143 -0.51428571 -0.5 -0.48571429 -0.47142857 -0.45714286 -0.44285714 -0.42857143 -0.41428571 -0.4 -0.38571429 -0.37142857 -0.35714286 -0.34285714 -0.32857143 -0.31428571 -0.3 -0.28571429 -0.27142857 -0.25714286 -0.24285714 -0.22857143 -0.21428571 -0.2 -0.18571429 -0.17142857 -0.15714286 -0.14285714 -0.12857143 -0.11428571 -0.1 -0.08571429 -0.07142857 -0.05714286 -0.04285714 -0.02857143 -0.01428571 0 0 0 0 0 0
  line L23 (-10.4811, 4.1595) -> (-9.7605, 3.8729)
  arc A47 (-9.1699, 2.6646) -> (-9.7605, 3.8729) centre (-10.1302, 2.9437) ccw
  circle A48 centre (0, 0) radius 2.5
  circle A49 centre (0, 0) radius 9.5492
  circle A50 centre (0, 0) radius 15.4387
  line L24 (6.8926, -6.609) -> (10.9038, -10.9299)
  line L25 (-2.6646, 9.1699) -> (-4.5624, 14.7492)
  constraint concentric A0 A49
  constraint coincident A16.end A49
  constraint concentric A49 A50
  constraint coincident A20.end A21.end
  constraint coincident A50 L24.end
  constraint coincident A40.end A41.end
  constraint coincident A50 L25.end
extrude "Extrude3" cut sketch "Sketch1 (2)" against normal blind 8 contours A21 L10 S10 A22 S11 L11 A23 A24 A25 L12 S12 A26 S13 L13 A27 A28 A29 L14 S14 A30 S15 L15 A31 A32 A33 L16 S16 A34 S17 L17 A35 A36 A37 L18 S18 A38 S19 L19 A39 A40 A49 A50 L24 L25 | A37 L18 S18 A38 S19 L19 A39 A49 | A33 L16 S16 A34 S17 L17 A35 A49 | A21 L10 S10 A22 S11 L11 A23 A49 | A29 L14 S14 A30 S15 L15 A31 A49 | A25 L12 S12 A26 S13 L13 A27 A49 in component "Spur Gear (12 teeth)"
sketch "Sketch2 (2)" plane through (-81.2627, 96.8451, -716.9768) normal (0.111619, -0.133022, 0.984808) x (0.766044, 0.642788, 0)
  arc A0 (-12.2773, -144.5539) -> (-12.2773, -163.1013) centre (-10, -153.8276) ccw
  arc A1 (-11.5263, -164.2169) -> (-12.2773, -163.1013) centre (-12.5158, -164.0724) ccw
  line L0 (-11.5263, -164.2169) -> (-11.6383, -164.9843)
  spline S0 degree 5 poles (-11.6383, -164.9843) (-11.6395, -164.9923) (-11.6416, -165.0083) (-11.6439, -165.0324) (-11.6456, -165.0646) (-11.6458, -165.105) (-11.6445, -165.1456) (-11.6423, -165.1863) (-11.6396, -165.227) (-11.6366, -165.2678) (-11.6333, -165.3085) (-11.6295, -165.3494) (-11.625, -165.3902) (-11.6199, -165.4311) (-11.614, -165.4721) (-11.6075, -165.513) (-11.6005, -165.554) (-11.5929, -165.595) (-11.585, -165.636) (-11.5766, -165.6771) (-11.5678, -165.7181) (-11.5587, -165.7591) (-11.5491, -165.8001) (-11.539, -165.8411) (-11.5285, -165.8822) (-11.5175, -165.9232) (-11.5062, -165.9642) (-11.4944, -166.0052) (-11.4823, -166.0462) (-11.4698, -166.0872) (-11.4569, -166.1281) (-11.4437, -166.1691) (-11.4301, -166.21) (-11.4161, -166.2509) (-11.4018, -166.2918) (-11.3871, -166.3326) (-11.372, -166.3734) (-11.3566, -166.4142) (-11.3409, -166.455) (-11.3248, -166.4958) (-11.3084, -166.5365) (-11.2917, -166.5771) (-11.2746, -166.6178) (-11.2572, -166.6584) (-11.2395, -166.6989) (-11.2215, -166.7395) (-11.2031, -166.78) (-11.1844, -166.8204) (-11.1654, -166.8608) (-11.1461, -166.9011) (-11.1265, -166.9415) (-11.1066, -166.9817) (-11.0863, -167.0219) (-11.0658, -167.0621) (-11.045, -167.1022) (-11.0239, -167.1422) (-11.0024, -167.1822) (-10.9807, -167.2222) (-10.9587, -167.2621) (-10.9364, -167.3019) (-10.9138, -167.3417) (-10.8909, -167.3814) (-10.8678, -167.421) (-10.8443, -167.4606) (-10.8206, -167.5001) (-10.7966, -167.5396) (-10.7723, -167.579) (-10.7477, -167.6183) (-10.7229, -167.6576) (-10.6978, -167.6967) (-10.6724, -167.7359) (-10.6518, -167.7671) (-10.6363, -167.7905) (-10.6259, -167.8061) (-10.6207, -167.8139) knots 0 0 0 0 0 0 0.01428571 0.02857143 0.04285714 0.05714286 0.07142857 0.08571429 0.1 0.11428571 0.12857143 0.14285714 0.15714286 0.17142857 0.18571429 0.2 0.21428571 0.22857143 0.24285714 0.25714286 0.27142857 0.28571429 0.3 0.31428571 0.32857143 0.34285714 0.35714286 0.37142857 0.38571429 0.4 0.41428571 0.42857143 0.44285714 0.45714286 0.47142857 0.48571429 0.5 0.51428571 0.52857143 0.54285714 0.55714286 0.57142857 0.58571429 0.6 0.61428571 0.62857143 0.64285714 0.65714286 0.67142857 0.68571429 0.7 0.71428571 0.72857143 0.74285714 0.75714286 0.77142857 0.78571429 0.8 0.81428571 0.82857143 0.84285714 0.85714286 0.87142857 0.88571429 0.9 0.91428571 0.92857143 0.94285714 0.95714286 0.97142857 0.98571429 1 1 1 1 1 1
  arc A2 (-10.6207, -167.8139) -> (-9.3793, -167.8139) centre (-10, -153.8276) ccw
  spline S1 degree 5 poles (-9.3793, -167.8139) (-9.3741, -167.8061) (-9.3637, -167.7905) (-9.3482, -167.7671) (-9.3276, -167.7359) (-9.3022, -167.6967) (-9.2771, -167.6576) (-9.2523, -167.6183) (-9.2277, -167.579) (-9.2034, -167.5396) (-9.1794, -167.5001) (-9.1557, -167.4606) (-9.1322, -167.421) (-9.1091, -167.3814) (-9.0862, -167.3417) (-9.0636, -167.3019) (-9.0413, -167.2621) (-9.0193, -167.2222) (-8.9976, -167.1822) (-8.9761, -167.1422) (-8.955, -167.1022) (-8.9342, -167.0621) (-8.9137, -167.0219) (-8.8934, -166.9817) (-8.8735, -166.9415) (-8.8539, -166.9011) (-8.8346, -166.8608) (-8.8156, -166.8204) (-8.7969, -166.78) (-8.7785, -166.7395) (-8.7605, -166.6989) (-8.7428, -166.6584) (-8.7254, -166.6178) (-8.7083, -166.5771) (-8.6916, -166.5365) (-8.6752, -166.4958) (-8.6591, -166.455) (-8.6434, -166.4142) (-8.628, -166.3734) (-8.6129, -166.3326) (-8.5982, -166.2918) (-8.5839, -166.2509) (-8.5699, -166.21) (-8.5563, -166.1691) (-8.5431, -166.1281) (-8.5302, -166.0872) (-8.5177, -166.0462) (-8.5056, -166.0052) (-8.4938, -165.9642) (-8.4825, -165.9232) (-8.4715, -165.8822) (-8.461, -165.8411) (-8.4509, -165.8001) (-8.4413, -165.7591) (-8.4322, -165.7181) (-8.4234, -165.6771) (-8.415, -165.636) (-8.4071, -165.595) (-8.3995, -165.554) (-8.3925, -165.513) (-8.386, -165.4721) (-8.3801, -165.4311) (-8.375, -165.3902) (-8.3705, -165.3494) (-8.3667, -165.3085) (-8.3634, -165.2678) (-8.3604, -165.227) (-8.3577, -165.1863) (-8.3555, -165.1456) (-8.3542, -165.105) (-8.3544, -165.0646) (-8.3561, -165.0324) (-8.3584, -165.0083) (-8.3605, -164.9923) (-8.3617, -164.9843) knots -1 -1 -1 -1 -1 -1 -0.98571429 -0.97142857 -0.95714286 -0.94285714 -0.92857143 -0.91428571 -0.9 -0.88571429 -0.87142857 -0.85714286 -0.84285714 -0.82857143 -0.81428571 -0.8 -0.78571429 -0.77142857 -0.75714286 -0.74285714 -0.72857143 -0.71428571 -0.7 -0.68571429 -0.67142857 -0.65714286 -0.64285714 -0.62857143 -0.61428571 -0.6 -0.58571429 -0.57142857 -0.55714286 -0.54285714 -0.52857143 -0.51428571 -0.5 -0.48571429 -0.47142857 -0.45714286 -0.44285714 -0.42857143 -0.41428571 -0.4 -0.38571429 -0.37142857 -0.35714286 -0.34285714 -0.32857143 -0.31428571 -0.3 -0.28571429 -0.27142857 -0.25714286 -0.24285714 -0.22857143 -0.21428571 -0.2 -0.18571429 -0.17142857 -0.15714286 -0.14285714 -0.12857143 -0.11428571 -0.1 -0.08571429 -0.07142857 -0.05714286 -0.04285714 -0.02857143 -0.01428571 0 0 0 0 0 0
  line L1 (-8.3617, -164.9843) -> (-8.4737, -164.2169)
  arc A3 (-7.7227, -163.1013) -> (-8.4737, -164.2169) centre (-7.4842, -164.0724) ccw
  arc A4 (-7.7227, -163.1013) -> (-7.3354, -162.9975) centre (-10, -153.8276) ccw
  arc A5 (-6.1271, -163.5882) -> (-7.3354, -162.9975) centre (-7.0563, -163.9578) ccw
  line L2 (-6.1271, -163.5882) -> (-5.8405, -164.3087)
  spline S2 degree 5 poles (-5.8405, -164.3087) (-5.8375, -164.3162) (-5.8313, -164.3311) (-5.8213, -164.3532) (-5.8067, -164.3819) (-5.7866, -164.417) (-5.7651, -164.4515) (-5.7429, -164.4856) (-5.7203, -164.5196) (-5.6973, -164.5534) (-5.674, -164.587) (-5.6503, -164.6205) (-5.626, -164.6537) (-5.6011, -164.6865) (-5.5756, -164.719) (-5.5495, -164.7513) (-5.5228, -164.7832) (-5.4958, -164.8149) (-5.4684, -164.8465) (-5.4407, -164.8778) (-5.4126, -164.909) (-5.3841, -164.9399) (-5.3553, -164.9706) (-5.326, -165.0011) (-5.2964, -165.0314) (-5.2664, -165.0614) (-5.2361, -165.0913) (-5.2054, -165.1209) (-5.1744, -165.1504) (-5.1431, -165.1796) (-5.1115, -165.2086) (-5.0796, -165.2375) (-5.0473, -165.2661) (-5.0148, -165.2945) (-4.9819, -165.3228) (-4.9488, -165.3508) (-4.9153, -165.3786) (-4.8816, -165.4063) (-4.8476, -165.4337) (-4.8133, -165.461) (-4.7787, -165.488) (-4.7439, -165.5149) (-4.7088, -165.5415) (-4.6734, -165.568) (-4.6378, -165.5943) (-4.6019, -165.6203) (-4.5657, -165.6462) (-4.5293, -165.6719) (-4.4927, -165.6974) (-4.4558, -165.7227) (-4.4187, -165.7478) (-4.3813, -165.7727) (-4.3437, -165.7974) (-4.3058, -165.8219) (-4.2677, -165.8462) (-4.2294, -165.8703) (-4.1908, -165.8943) (-4.152, -165.918) (-4.113, -165.9415) (-4.0738, -165.9649) (-4.0344, -165.988) (-3.9947, -166.011) (-3.9548, -166.0337) (-3.9147, -166.0563) (-3.8744, -166.0787) (-3.8339, -166.1008) (-3.7931, -166.1228) (-3.7522, -166.1446) (-3.7111, -166.1661) (-3.6697, -166.1875) (-3.6282, -166.2087) (-3.5948, -166.2255) (-3.5696, -166.238) (-3.5528, -166.2463) (-3.5444, -166.2504) knots 0 0 0 0 0 0 0.01428571 0.02857143 0.04285714 0.05714286 0.07142857 0.08571429 0.1 0.11428571 0.12857143 0.14285714 0.15714286 0.17142857 0.18571429 0.2 0.21428571 0.22857143 0.24285714 0.25714286 0.27142857 0.28571429 0.3 0.31428571 0.32857143 0.34285714 0.35714286 0.37142857 0.38571429 0.4 0.41428571 0.42857143 0.44285714 0.45714286 0.47142857 0.48571429 0.5 0.51428571 0.52857143 0.54285714 0.55714286 0.57142857 0.58571429 0.6 0.61428571 0.62857143 0.64285714 0.65714286 0.67142857 0.68571429 0.7 0.71428571 0.72857143 0.74285714 0.75714286 0.77142857 0.78571429 0.8 0.81428571 0.82857143 0.84285714 0.85714286 0.87142857 0.88571429 0.9 0.91428571 0.92857143 0.94285714 0.95714286 0.97142857 0.98571429 1 1 1 1 1 1
  arc A6 (-3.5444, -166.2504) -> (-2.4693, -165.6297) centre (-10, -153.8276) ccw
  spline S3 degree 5 poles (-2.4693, -165.6297) (-2.4687, -165.6204) (-2.4675, -165.6017) (-2.4658, -165.5736) (-2.4636, -165.5363) (-2.4612, -165.4898) (-2.459, -165.4433) (-2.4571, -165.3968) (-2.4555, -165.3505) (-2.4542, -165.3042) (-2.4531, -165.2581) (-2.4523, -165.212) (-2.4518, -165.166) (-2.4516, -165.1201) (-2.4516, -165.0742) (-2.4519, -165.0285) (-2.4525, -164.9828) (-2.4534, -164.9373) (-2.4546, -164.8918) (-2.456, -164.8465) (-2.4577, -164.8012) (-2.4597, -164.7561) (-2.462, -164.711) (-2.4646, -164.6661) (-2.4675, -164.6213) (-2.4707, -164.5766) (-2.4741, -164.532) (-2.4779, -164.4875) (-2.4819, -164.4431) (-2.4863, -164.3989) (-2.4909, -164.3548) (-2.4958, -164.3108) (-2.5011, -164.2669) (-2.5066, -164.2232) (-2.5124, -164.1796) (-2.5186, -164.1361) (-2.525, -164.0928) (-2.5318, -164.0496) (-2.5389, -164.0066) (-2.5462, -163.9637) (-2.5539, -163.921) (-2.562, -163.8784) (-2.5703, -163.836) (-2.579, -163.7938) (-2.588, -163.7517) (-2.5973, -163.7098) (-2.607, -163.6681) (-2.617, -163.6265) (-2.6273, -163.5851) (-2.638, -163.5439) (-2.649, -163.5029) (-2.6604, -163.4621) (-2.6722, -163.4216) (-2.6844, -163.3812) (-2.697, -163.3411) (-2.7099, -163.3012) (-2.7232, -163.2615) (-2.7368, -163.222) (-2.7508, -163.1828) (-2.7651, -163.1437) (-2.78, -163.105) (-2.7954, -163.0666) (-2.8114, -163.0286) (-2.828, -162.991) (-2.8451, -162.9538) (-2.8626, -162.9168) (-2.8804, -162.88) (-2.8984, -162.8434) (-2.9169, -162.8071) (-2.936, -162.7713) (-2.9564, -162.7363) (-2.9739, -162.7093) (-2.988, -162.6896) (-2.9978, -162.6768) (-3.0028, -162.6704) knots -1 -1 -1 -1 -1 -1 -0.98571429 -0.97142857 -0.95714286 -0.94285714 -0.92857143 -0.91428571 -0.9 -0.88571429 -0.87142857 -0.85714286 -0.84285714 -0.82857143 -0.81428571 -0.8 -0.78571429 -0.77142857 -0.75714286 -0.74285714 -0.72857143 -0.71428571 -0.7 -0.68571429 -0.67142857 -0.65714286 -0.64285714 -0.62857143 -0.61428571 -0.6 -0.58571429 -0.57142857 -0.55714286 -0.54285714 -0.52857143 -0.51428571 -0.5 -0.48571429 -0.47142857 -0.45714286 -0.44285714 -0.42857143 -0.41428571 -0.4 -0.38571429 -0.37142857 -0.35714286 -0.34285714 -0.32857143 -0.31428571 -0.3 -0.28571429 -0.27142857 -0.25714286 -0.24285714 -0.22857143 -0.21428571 -0.2 -0.18571429 -0.17142857 -0.15714286 -0.14285714 -0.12857143 -0.11428571 -0.1 -0.08571429 -0.07142857 -0.05714286 -0.04285714 -0.02857143 -0.01428571 0 0 0 0 0 0
  line L3 (-3.0028, -162.6704) -> (-3.4836, -162.0619)
  arc A7 (-3.391, -160.7202) -> (-3.4836, -162.0619) centre (-2.6989, -161.442) ccw
  arc A8 (-3.391, -160.7202) -> (-3.1074, -160.4367) centre (-10, -153.8276) ccw
  arc A9 (-1.7657, -160.3441) -> (-3.1074, -160.4367) centre (-2.3856, -161.1288) ccw
  line L4 (-1.7657, -160.3441) -> (-1.1572, -160.8248)
  spline S4 degree 5 poles (-1.1572, -160.8248) (-1.1509, -160.8298) (-1.138, -160.8396) (-1.1184, -160.8537) (-1.0913, -160.8713) (-1.0563, -160.8916) (-1.0206, -160.9108) (-0.9843, -160.9292) (-0.9477, -160.9473) (-0.9109, -160.965) (-0.8739, -160.9825) (-0.8366, -160.9996) (-0.799, -161.0162) (-0.761, -161.0322) (-0.7226, -161.0476) (-0.6839, -161.0625) (-0.6449, -161.0769) (-0.6056, -161.0908) (-0.5661, -161.1044) (-0.5264, -161.1177) (-0.4865, -161.1306) (-0.4464, -161.1432) (-0.406, -161.1554) (-0.3655, -161.1672) (-0.3247, -161.1786) (-0.2837, -161.1896) (-0.2425, -161.2003) (-0.2011, -161.2106) (-0.1596, -161.2206) (-0.1178, -161.2303) (-0.0759, -161.2396) (-0.0338, -161.2486) (0.0084, -161.2573) (0.0508, -161.2656) (0.0934, -161.2737) (0.1361, -161.2814) (0.179, -161.2888) (0.222, -161.2958) (0.2652, -161.3026) (0.3085, -161.309) (0.352, -161.3152) (0.3956, -161.321) (0.4393, -161.3266) (0.4832, -161.3318) (0.5271, -161.3367) (0.5713, -161.3414) (0.6155, -161.3457) (0.6599, -161.3497) (0.7044, -161.3535) (0.7489, -161.3569) (0.7937, -161.3601) (0.8385, -161.363) (0.8834, -161.3656) (0.9285, -161.3679) (0.9736, -161.3699) (1.0189, -161.3716) (1.0642, -161.3731) (1.1097, -161.3742) (1.1552, -161.3751) (1.2009, -161.3757) (1.2466, -161.376) (1.2924, -161.3761) (1.3384, -161.3758) (1.3844, -161.3753) (1.4305, -161.3745) (1.4766, -161.3735) (1.5229, -161.3721) (1.5692, -161.3705) (1.6156, -161.3686) (1.6621, -161.3665) (1.7087, -161.364) (1.746, -161.3619) (1.774, -161.3601) (1.7927, -161.3589) (1.8021, -161.3583) knots 0 0 0 0 0 0 0.01428571 0.02857143 0.04285714 0.05714286 0.07142857 0.08571429 0.1 0.11428571 0.12857143 0.14285714 0.15714286 0.17142857 0.18571429 0.2 0.21428571 0.22857143 0.24285714 0.25714286 0.27142857 0.28571429 0.3 0.31428571 0.32857143 0.34285714 0.35714286 0.37142857 0.38571429 0.4 0.41428571 0.42857143 0.44285714 0.45714286 0.47142857 0.48571429 0.5 0.51428571 0.52857143 0.54285714 0.55714286 0.57142857 0.58571429 0.6 0.61428571 0.62857143 0.64285714 0.65714286 0.67142857 0.68571429 0.7 0.71428571 0.72857143 0.74285714 0.75714286 0.77142857 0.78571429 0.8 0.81428571 0.82857143 0.84285714 0.85714286 0.87142857 0.88571429 0.9 0.91428571 0.92857143 0.94285714 0.95714286 0.97142857 0.98571429 1 1 1 1 1 1
  arc A10 (1.8021, -161.3583) -> (2.4228, -160.2832) centre (-10, -153.8276) ccw
  spline S5 degree 5 poles (2.4228, -160.2832) (2.4186, -160.2748) (2.4104, -160.258) (2.3979, -160.2329) (2.3811, -160.1995) (2.3599, -160.1579) (2.3385, -160.1166) (2.3169, -160.0754) (2.2952, -160.0345) (2.2732, -159.9938) (2.251, -159.9532) (2.2287, -159.9129) (2.2061, -159.8728) (2.1834, -159.8329) (2.1604, -159.7933) (2.1373, -159.7538) (2.1139, -159.7146) (2.0904, -159.6756) (2.0667, -159.6368) (2.0427, -159.5982) (2.0186, -159.5599) (1.9943, -159.5218) (1.9698, -159.484) (1.9451, -159.4463) (1.9202, -159.409) (1.8951, -159.3718) (1.8698, -159.3349) (1.8443, -159.2983) (1.8186, -159.2619) (1.7927, -159.2257) (1.7666, -159.1898) (1.7404, -159.1542) (1.7139, -159.1188) (1.6873, -159.0837) (1.6604, -159.0489) (1.6334, -159.0143) (1.6061, -158.9801) (1.5787, -158.946) (1.551, -158.9123) (1.5232, -158.8789) (1.4952, -158.8457) (1.4669, -158.8129) (1.4385, -158.7803) (1.4099, -158.7481) (1.381, -158.7161) (1.352, -158.6845) (1.3227, -158.6532) (1.2933, -158.6222) (1.2637, -158.5915) (1.2338, -158.5612) (1.2038, -158.5312) (1.1735, -158.5016) (1.143, -158.4723) (1.1123, -158.4435) (1.0814, -158.415) (1.0502, -158.387) (1.0189, -158.3592) (0.9873, -158.3318) (0.9556, -158.3048) (0.9236, -158.2782) (0.8914, -158.2521) (0.8589, -158.2265) (0.826, -158.2016) (0.7929, -158.1773) (0.7594, -158.1536) (0.7258, -158.1303) (0.692, -158.1073) (0.658, -158.0847) (0.6239, -158.0625) (0.5894, -158.0411) (0.5543, -158.021) (0.5256, -158.0063) (0.5035, -157.9963) (0.4886, -157.9901) (0.4811, -157.9871) knots -1 -1 -1 -1 -1 -1 -0.98571429 -0.97142857 -0.95714286 -0.94285714 -0.92857143 -0.91428571 -0.9 -0.88571429 -0.87142857 -0.85714286 -0.84285714 -0.82857143 -0.81428571 -0.8 -0.78571429 -0.77142857 -0.75714286 -0.74285714 -0.72857143 -0.71428571 -0.7 -0.68571429 -0.67142857 -0.65714286 -0.64285714 -0.62857143 -0.61428571 -0.6 -0.58571429 -0.57142857 -0.55714286 -0.54285714 -0.52857143 -0.51428571 -0.5 -0.48571429 -0.47142857 -0.45714286 -0.44285714 -0.42857143 -0.41428571 -0.4 -0.38571429 -0.37142857 -0.35714286 -0.34285714 -0.32857143 -0.31428571 -0.3 -0.28571429 -0.27142857 -0.25714286 -0.24285714 -0.22857143 -0.21428571 -0.2 -0.18571429 -0.17142857 -0.15714286 -0.14285714 -0.12857143 -0.11428571 -0.1 -0.08571429 -0.07142857 -0.05714286 -0.04285714 -0.02857143 -0.01428571 0 0 0 0 0 0
  line L5 (0.4811, -157.9871) -> (-0.2395, -157.7005)
  arc A11 (-0.8301, -156.4923) -> (-0.2395, -157.7005) centre (0.1302, -156.7713) ccw
  arc A12 (-0.8301, -156.4923) -> (-0.7263, -156.1049) centre (-10, -153.8276) ccw
  arc A13 (0.3893, -155.3539) -> (-0.7263, -156.1049) centre (0.2448, -156.3434) ccw
  line L6 (0.3893, -155.3539) -> (1.1567, -155.4659)
  spline S6 degree 5 poles (1.1567, -155.4659) (1.1647, -155.4671) (1.1807, -155.4692) (1.2048, -155.4715) (1.237, -155.4732) (1.2774, -155.4734) (1.318, -155.4721) (1.3587, -155.4699) (1.3994, -155.4672) (1.4401, -155.4642) (1.4809, -155.4609) (1.5218, -155.4571) (1.5626, -155.4526) (1.6035, -155.4475) (1.6445, -155.4417) (1.6854, -155.4351) (1.7264, -155.4281) (1.7674, -155.4205) (1.8084, -155.4126) (1.8494, -155.4042) (1.8905, -155.3955) (1.9315, -155.3863) (1.9725, -155.3767) (2.0135, -155.3666) (2.0545, -155.3561) (2.0956, -155.3451) (2.1366, -155.3338) (2.1776, -155.322) (2.2186, -155.3099) (2.2595, -155.2974) (2.3005, -155.2845) (2.3414, -155.2713) (2.3824, -155.2577) (2.4233, -155.2437) (2.4641, -155.2294) (2.505, -155.2147) (2.5458, -155.1997) (2.5866, -155.1843) (2.6274, -155.1685) (2.6681, -155.1525) (2.7088, -155.1361) (2.7495, -155.1193) (2.7902, -155.1022) (2.8308, -155.0848) (2.8713, -155.0671) (2.9119, -155.0491) (2.9523, -155.0307) (2.9928, -155.012) (3.0332, -154.993) (3.0735, -154.9737) (3.1138, -154.9541) (3.1541, -154.9342) (3.1943, -154.914) (3.2345, -154.8934) (3.2746, -154.8726) (3.3146, -154.8515) (3.3546, -154.8301) (3.3946, -154.8083) (3.4344, -154.7863) (3.4743, -154.764) (3.514, -154.7414) (3.5538, -154.7185) (3.5934, -154.6954) (3.633, -154.6719) (3.6725, -154.6482) (3.712, -154.6242) (3.7514, -154.5999) (3.7907, -154.5753) (3.8299, -154.5505) (3.8691, -154.5254) (3.9082, -154.5) (3.9395, -154.4795) (3.9629, -154.4639) (3.9784, -154.4535) (3.9862, -154.4483) knots 0 0 0 0 0 0 0.01428571 0.02857143 0.04285714 0.05714286 0.07142857 0.08571429 0.1 0.11428571 0.12857143 0.14285714 0.15714286 0.17142857 0.18571429 0.2 0.21428571 0.22857143 0.24285714 0.25714286 0.27142857 0.28571429 0.3 0.31428571 0.32857143 0.34285714 0.35714286 0.37142857 0.38571429 0.4 0.41428571 0.42857143 0.44285714 0.45714286 0.47142857 0.48571429 0.5 0.51428571 0.52857143 0.54285714 0.55714286 0.57142857 0.58571429 0.6 0.61428571 0.62857143 0.64285714 0.65714286 0.67142857 0.68571429 0.7 0.71428571 0.72857143 0.74285714 0.75714286 0.77142857 0.78571429 0.8 0.81428571 0.82857143 0.84285714 0.85714286 0.87142857 0.88571429 0.9 0.91428571 0.92857143 0.94285714 0.95714286 0.97142857 0.98571429 1 1 1 1 1 1
  arc A14 (3.9862, -154.4483) -> (3.9862, -153.2069) centre (-10, -153.8276) ccw
  spline S7 degree 5 poles (3.9862, -153.2069) (3.9784, -153.2017) (3.9629, -153.1913) (3.9395, -153.1758) (3.9082, -153.1553) (3.8691, -153.1299) (3.8299, -153.1047) (3.7907, -153.0799) (3.7514, -153.0553) (3.712, -153.031) (3.6725, -153.007) (3.633, -152.9833) (3.5934, -152.9599) (3.5538, -152.9367) (3.514, -152.9138) (3.4743, -152.8912) (3.4344, -152.8689) (3.3946, -152.8469) (3.3546, -152.8252) (3.3146, -152.8038) (3.2746, -152.7826) (3.2345, -152.7618) (3.1943, -152.7413) (3.1541, -152.721) (3.1138, -152.7011) (3.0735, -152.6815) (3.0332, -152.6622) (2.9928, -152.6432) (2.9523, -152.6245) (2.9119, -152.6062) (2.8713, -152.5881) (2.8308, -152.5704) (2.7902, -152.553) (2.7495, -152.5359) (2.7088, -152.5192) (2.6681, -152.5028) (2.6274, -152.4867) (2.5866, -152.471) (2.5458, -152.4556) (2.505, -152.4405) (2.4641, -152.4258) (2.4233, -152.4115) (2.3824, -152.3975) (2.3414, -152.3839) (2.3005, -152.3707) (2.2595, -152.3578) (2.2186, -152.3453) (2.1776, -152.3332) (2.1366, -152.3215) (2.0956, -152.3101) (2.0545, -152.2991) (2.0135, -152.2886) (1.9725, -152.2786) (1.9315, -152.2689) (1.8905, -152.2598) (1.8494, -152.251) (1.8084, -152.2427) (1.7674, -152.2347) (1.7264, -152.2272) (1.6854, -152.2201) (1.6445, -152.2136) (1.6035, -152.2077) (1.5626, -152.2026) (1.5218, -152.1982) (1.4809, -152.1943) (1.4401, -152.191) (1.3994, -152.188) (1.3587, -152.1853) (1.318, -152.1832) (1.2774, -152.1819) (1.237, -152.182) (1.2048, -152.1837) (1.1807, -152.1861) (1.1647, -152.1881) (1.1567, -152.1893) knots -1 -1 -1 -1 -1 -1 -0.98571429 -0.97142857 -0.95714286 -0.94285714 -0.92857143 -0.91428571 -0.9 -0.88571429 -0.87142857 -0.85714286 -0.84285714 -0.82857143 -0.81428571 -0.8 -0.78571429 -0.77142857 -0.75714286 -0.74285714 -0.72857143 -0.71428571 -0.7 -0.68571429 -0.67142857 -0.65714286 -0.64285714 -0.62857143 -0.61428571 -0.6 -0.58571429 -0.57142857 -0.55714286 -0.54285714 -0.52857143 -0.51428571 -0.5 -0.48571429 -0.47142857 -0.45714286 -0.44285714 -0.42857143 -0.41428571 -0.4 -0.38571429 -0.37142857 -0.35714286 -0.34285714 -0.32857143 -0.31428571 -0.3 -0.28571429 -0.27142857 -0.25714286 -0.24285714 -0.22857143 -0.21428571 -0.2 -0.18571429 -0.17142857 -0.15714286 -0.14285714 -0.12857143 -0.11428571 -0.1 -0.08571429 -0.07142857 -0.05714286 -0.04285714 -0.02857143 -0.01428571 0 0 0 0 0 0
  line L7 (1.1567, -152.1893) -> (0.3893, -152.3013)
  arc A15 (-0.7263, -151.5503) -> (0.3893, -152.3013) centre (0.2448, -151.3118) ccw
  arc A16 (-0.7263, -151.5503) -> (-0.8301, -151.163) centre (-10, -153.8276) ccw
  arc A17 (-0.2395, -149.9548) -> (-0.8301, -151.163) centre (0.1302, -150.8839) ccw
  line L8 (-0.2395, -149.9548) -> (0.4811, -149.6681)
  spline S8 degree 5 poles (0.4811, -149.6681) (0.4886, -149.6651) (0.5035, -149.6589) (0.5256, -149.6489) (0.5543, -149.6343) (0.5894, -149.6142) (0.6239, -149.5928) (0.658, -149.5706) (0.692, -149.5479) (0.7258, -149.5249) (0.7594, -149.5016) (0.7929, -149.4779) (0.826, -149.4536) (0.8589, -149.4287) (0.8914, -149.4032) (0.9236, -149.3771) (0.9556, -149.3505) (0.9873, -149.3234) (1.0189, -149.296) (1.0502, -149.2683) (1.0814, -149.2402) (1.1123, -149.2117) (1.143, -149.1829) (1.1735, -149.1537) (1.2038, -149.124) (1.2338, -149.094) (1.2637, -149.0637) (1.2933, -149.033) (1.3227, -149.002) (1.352, -148.9707) (1.381, -148.9391) (1.4099, -148.9072) (1.4385, -148.8749) (1.4669, -148.8424) (1.4952, -148.8095) (1.5232, -148.7764) (1.551, -148.7429) (1.5787, -148.7092) (1.6061, -148.6752) (1.6334, -148.6409) (1.6604, -148.6063) (1.6873, -148.5715) (1.7139, -148.5364) (1.7404, -148.501) (1.7666, -148.4654) (1.7927, -148.4295) (1.8186, -148.3934) (1.8443, -148.357) (1.8698, -148.3203) (1.8951, -148.2834) (1.9202, -148.2463) (1.9451, -148.2089) (1.9698, -148.1713) (1.9943, -148.1334) (2.0186, -148.0953) (2.0427, -148.057) (2.0667, -148.0184) (2.0904, -147.9797) (2.1139, -147.9407) (2.1373, -147.9014) (2.1604, -147.862) (2.1834, -147.8223) (2.2061, -147.7824) (2.2287, -147.7423) (2.251, -147.702) (2.2732, -147.6615) (2.2952, -147.6208) (2.3169, -147.5798) (2.3385, -147.5387) (2.3599, -147.4973) (2.3811, -147.4558) (2.3979, -147.4224) (2.4104, -147.3972) (2.4186, -147.3804) (2.4228, -147.372) knots 0 0 0 0 0 0 0.01428571 0.02857143 0.04285714 0.05714286 0.07142857 0.08571429 0.1 0.11428571 0.12857143 0.14285714 0.15714286 0.17142857 0.18571429 0.2 0.21428571 0.22857143 0.24285714 0.25714286 0.27142857 0.28571429 0.3 0.31428571 0.32857143 0.34285714 0.35714286 0.37142857 0.38571429 0.4 0.41428571 0.42857143 0.44285714 0.45714286 0.47142857 0.48571429 0.5 0.51428571 0.52857143 0.54285714 0.55714286 0.57142857 0.58571429 0.6 0.61428571 0.62857143 0.64285714 0.65714286 0.67142857 0.68571429 0.7 0.71428571 0.72857143 0.74285714 0.75714286 0.77142857 0.78571429 0.8 0.81428571 0.82857143 0.84285714 0.85714286 0.87142857 0.88571429 0.9 0.91428571 0.92857143 0.94285714 0.95714286 0.97142857 0.98571429 1 1 1 1 1 1
  arc A18 (2.4228, -147.372) -> (1.8021, -146.297) centre (-10, -153.8276) ccw